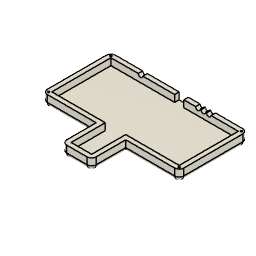
ControllerBottomHalf (Autodesk Fusion 360 design; units mm, degrees)
part number: 2026-04-19-10-27-17-976
Autodesk Fusion 360 part; units mm, degrees
sketch "Sketch1" plane through (0, 0, 0) normal (0, 1, 0) x (1, 0, 0)
  line L0 (0, 0) -> (300, 0)
  line L1 (300, 0) -> (300, -150)
  line L2 (300, -150) -> (0, -150)
  line L3 (0, -150) -> (0, 0)
  line L4 (150, -150) -> (117.5, -150)
  line L5 (150, -150) -> (182.5, -150)
  line L6 (117.5, -150) -> (117.5, -225)
  line L7 (182.5, -150) -> (182.5, -225)
  line L8 (117.5, -225) -> (182.5, -225)
  dimension "d1" = 300
  dimension "d2" = 150
  dimension "d3" = 32.5
  dimension "d4" = 32.5
  dimension "d5" = 75
  dimension "d6" = 75
  constraint horizontal L0
  constraint vertical L1
  constraint horizontal L2
  constraint vertical L3
  constraint coincident L0.start L3.end
  constraint midpoint L2 L4.start
  constraint parallel L2 L4
  constraint parallel L2 L5
  constraint perpendicular L2 L6
  constraint perpendicular L2 L7
  measures "d1" distance of L0.start L0.end
  measures "d2" distance of L0.start L2.end
  measures "d3" distance of L4.start L4.end
  measures "d4" distance of L4.start L5.end
  measures "d5" distance of L4.end L6.end
  measures "d6" distance of L5.end L7.end
extrude "Extrude1" add sketch "Sketch1" along normal blind 25
fillet "Fillet1" radius 10 6 edges at (117.5, 12.5, 225) (0, 12.5, 150) (0, 12.5, 0) (300, 12.5, 0) (300, 12.5, 150) (182.5, 12.5, 225) 1 faces at (139.1667, 0, 50)
shell "Shell1" thickness 10 removed faces 1 at (139.1667, 25, 50)
sketch "Sketch2" plane through (0, 0, 0) normal (0, 0, 1) x (1, 0, 0)
sketch "Sketch3" plane through (0, 25, 0) normal (0, 1, 0) x (-1, 0, 0)
  line L0 (-290, 10) -> (-290, 140)
  line L1 (-290, 140) -> (-172.5, 140)
  line L2 (-172.5, 140) -> (-172.5, 215)
  line L3 (-172.5, 215) -> (-127.5, 215)
  line L4 (-127.5, 215) -> (-127.5, 140)
  line L5 (-127.5, 140) -> (-10, 140)
  line L6 (-10, 140) -> (-10, 10)
  line L7 (-10, 10) -> (-290, 10)
  arc A0 (-117.5, 215) -> (-127.5, 225) centre (-127.5, 215) ccw
  line L8 (-127.5, 225) -> (-172.5, 225)
  arc A1 (-172.5, 225) -> (-182.5, 215) centre (-172.5, 215) ccw
  line L9 (-182.5, 215) -> (-182.5, 150)
  line L10 (-182.5, 150) -> (-290, 150)
  arc A2 (-290, 150) -> (-300, 140) centre (-290, 140) ccw
  line L11 (-300, 140) -> (-300, 10)
  arc A3 (-300, 10) -> (-290, 0) centre (-290, 10) ccw
  line L12 (-290, 0) -> (-10, 0)
  arc A4 (-10, 0) -> (0, 10) centre (-10, 10) ccw
  line L13 (0, 10) -> (0, 140)
  arc A5 (0, 140) -> (-10, 150) centre (-10, 140) ccw
  line L14 (-10, 150) -> (-117.5, 150)
  line L15 (-117.5, 150) -> (-117.5, 215)
  line L16 (-10, 140) -> (-2.9289, 147.0711)
  line L17 (-290, 140) -> (-297.0711, 147.0711)
  line L18 (-290, 10) -> (-297.0711, 2.9289)
  line L19 (-10, 10) -> (-2.9289, 2.9289)
  circle A6 centre (-293.5355, 143.5355) radius 2.116
  circle A7 centre (-293.5355, 6.4645) radius 2.116
  circle A8 centre (-6.4645, 6.4645) radius 2.116
  circle A9 centre (-6.4645, 143.5355) radius 2.116
  dimension "d12" = 4.232
  dimension "d13" = 4.232
  dimension "d14" = 4.232
  dimension "d15" = 4.232
  constraint coincident L5.end L6.start
  constraint midpoint A5 L16.end
  constraint coincident L0.end L1.start
  constraint midpoint A2 L17.end
  constraint coincident L0.start L7.end
  constraint midpoint A3 L18.end
  constraint coincident L6.end L7.start
  constraint midpoint A4 L19.end
  constraint midpoint L17 A6.centre
  constraint midpoint L18 A7.centre
  constraint midpoint L19 A8.centre
  constraint midpoint L16 A9.centre
  measures "d12" diameter of A6
  measures "d13" diameter of A7
  measures "d14" diameter of A8
  measures "d15" diameter of A9
hole "Hole1" at (293.5355, 25, 143.5355) at (293.5355, 25, 6.4645) at (6.4645, 25, 6.4645) at (6.4645, 25, 143.5355) direction (0, -1, 0) diameter 4.234 depth 8 tip angle 180
thread "Thread1" "ISO Metric profile 5.0 M5x0.8 M5x0.8 6H" thread offset 0 thread depth 7.4
sketch "Sketch4" plane through (0, 0, 0) normal (0, 0, -1) x (-1, 0, 0)
  line L0 (-10, 10) -> (-10, 25)
  line L1 (-10, 25) -> (-290, 25)
  line L2 (-290, 25) -> (-290, 10)
  line L3 (-290, 10) -> (-10, 10)
  line L4 (-10, 25) -> (-75, 25)
  circle A0 centre (-75, 25) radius 5
  line L5 (-290, 25) -> (-225, 25)
  circle A1 centre (-225, 25) radius 5
  line L6 (-220, 25) -> (-213, 25)
  circle A2 centre (-213, 25) radius 5
  line L7 (-208, 25) -> (-201, 25)
  circle A3 centre (-201, 25) radius 5
  dimension "d21" = 65
  dimension "d22" = 10
  dimension "d23" = 65
  dimension "d24" = 10
  dimension "d25" = 7
  dimension "d26" = 10
  dimension "d27" = 7
  dimension "d28" = 10
  constraint coincident L0.end L1.start
  constraint perpendicular L0 L4
  constraint coincident L4.end A0.centre
  constraint coincident L1.end L2.start
  constraint perpendicular L2 L5
  constraint coincident L5.end A1.centre
  constraint coincident A1 L6.start
  constraint coincident L1 L6.start
  constraint parallel L1 L6
  constraint coincident L6.end A2.centre
  constraint horizontal L7
  constraint coincident A2 L7.start
  constraint coincident L1 L7.start
  constraint coincident L7.end A3.centre
  measures "d21" distance of L0.end L4.end
  measures "d22" diameter of A0
  measures "d23" distance of L1.end L5.end
  measures "d24" diameter of A1
  measures "d25" distance of L6.start L6.end
  measures "d26" diameter of A2
  measures "d27" distance of L7.start L7.end
  measures "d28" diameter of A3
extrude "Extrude2" cut sketch "Sketch4" against normal blind 25 contours L1 L4 A0 | L1 L5 A1 | L1 L7 A3 | L1 L6 A2 picked at (-71.6853, 24.7516) picked at (-221.6853, 24.7516) picked at (-201, 21.676) picked at (-209.6853, 24.7516)
sketch "Sketch5" plane through (0, 0, 0) normal (0, 0, -1) x (-1, 0, 0)
  arc A0 (-218, 25) -> (-208, 25) centre (-213, 25) ccw
  line L0 (-218, 25) -> (-220, 25)
  arc A1 (-230, 25) -> (-220, 25) centre (-225, 25) ccw
  line L1 (-230, 25) -> (-290, 25)
  line L2 (-290, 25) -> (-290, 10)
  line L3 (-290, 10) -> (-10, 10)
  line L4 (-10, 10) -> (-10, 25)
  line L5 (-10, 25) -> (-70, 25)
  arc A2 (-80, 25) -> (-70, 25) centre (-75, 25) ccw
  line L6 (-80, 25) -> (-196, 25)
  arc A3 (-206, 25) -> (-196, 25) centre (-201, 25) ccw
  line L7 (-206, 25) -> (-208, 25)
  line L8 (-290, 25) -> (-166, 25)
  line L9 (-170, 25) -> (-150, 25)
  line L10 (-150, 25) -> (-150, 10)
  line L11 (-150, 10) -> (-170, 10)
  line L12 (-170, 10) -> (-170, 25)
  dimension "d31" = 124
  constraint coincident L1.end L2.start
  constraint perpendicular L2 L8
  constraint horizontal L9
  constraint vertical L10
  constraint horizontal L11
  constraint vertical L12
  constraint midpoint L3 L10.end
  constraint coincident L6 L9.start
  measures "d31" distance of L1.end L8.end
extrude "Extrude3" cut sketch "Sketch5" against normal blind 25 contours L3 L6 L8 L9 L10 L11 L12
